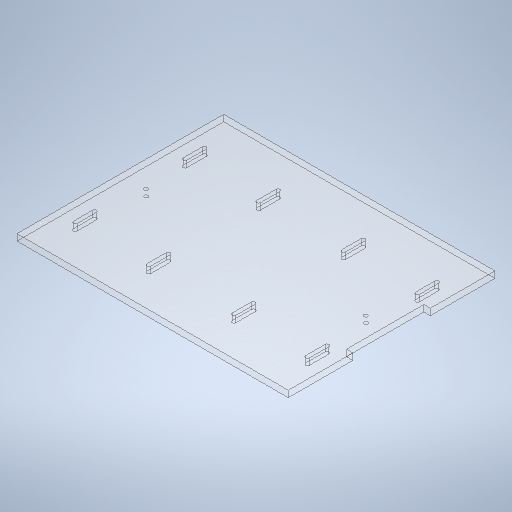
# Autodesk Inventor part: base_2
Saved by Autodesk Inventor 2025.3 (Build 293356030, 356C)
## iProperties
Created: 2026-06-26
Part Number: base_2
Material: Acrylic
Document SubType Name: Modeling
Designer: user
Density: 1.188 g/cm^3
Appearance: Transparent - Clear
Author: user
Autodesk Inventor part; units mm, degrees
ref_plane "YZ Plane" through (0, 0, 0) normal (1, 0, 0) x (0, 1, 0)
ref_plane "XZ Plane" through (0, 0, 0) normal (0, 1, 0) x (-1, 0, 0)
ref_plane "XY Plane" through (0, 0, 0) normal (0, 0, 1) x (1, 0, 0)
sketch "Sketch1" plane through (0, 0, 0) normal (0, 1, 0) x (-1, 0, 0)
  line L0 (0, 0) -> (-210, 0)
  line L1 (-210, 0) -> (-210, -160)
  line L2 (-210, -160) -> (0, -160)
  line L3 (75, -80) -> (-210, -80) construction
  line L4 (-105, 0) -> (-105, -160) construction
  line L5 (-43.5, 0) -> (-43.5, -160) construction
  line L6 (-133, 0) -> (-133, -160) construction
  line L7 (-15, -130) -> (-15, -115) construction
  line L8 (-15, -130) -> (-15, -115) construction
  line L9 (-13.5, -130) -> (-13.5, -115)
  line L10 (-16.5, -115) -> (-16.5, -130)
  arc A0 (-16.5, -130) -> (-13.5, -130) centre (-15, -130) ccw
  arc A1 (-13.5, -115) -> (-16.5, -115) centre (-15, -115) ccw
  line L11 (-72, -130) -> (-72, -115) construction
  line L12 (-72, -130) -> (-72, -115) construction
  line L13 (-73.5, -130) -> (-73.5, -115)
  line L14 (-70.5, -115) -> (-70.5, -130)
  arc A2 (-73.5, -130) -> (-70.5, -130) centre (-72, -130) ccw
  arc A3 (-70.5, -115) -> (-73.5, -115) centre (-72, -115) ccw
  line L15 (-125, -160) -> (-85, -160)
  line L16 (-85, -160) -> (-85, -155)
  line L17 (-85, -155) -> (-125, -155)
  line L18 (-125, -155) -> (-125, -160)
  line L19 (-195, -130) -> (-195, -115) construction
  line L20 (-195, -130) -> (-195, -115) construction
  line L21 (-196.5, -130) -> (-196.5, -115)
  line L22 (-193.5, -115) -> (-193.5, -130)
  arc A4 (-196.5, -130) -> (-193.5, -130) centre (-195, -130) ccw
  arc A5 (-193.5, -115) -> (-196.5, -115) centre (-195, -115) ccw
  line L23 (-139.5, -115) -> (-139.5, -130)
  line L24 (-138, -130) -> (-138, -115) construction
  line L25 (-136.5, -130) -> (-136.5, -115)
  arc A6 (-139.5, -130) -> (-136.5, -130) centre (-138, -130) ccw
  line L26 (-138, -130) -> (-138, -115) construction
  arc A7 (-136.5, -115) -> (-139.5, -115) centre (-138, -115) ccw
  line L27 (-105, -160) -> (-105, 0) construction
  line L28 (-15, -30) -> (-15, -45) construction
  line L29 (-15, -30) -> (-15, -45) construction
  line L30 (-13.5, -30) -> (-13.5, -45)
  line L31 (-16.5, -45) -> (-16.5, -30)
  arc A8 (-13.5, -30) -> (-16.5, -30) centre (-15, -30) ccw
  arc A9 (-16.5, -45) -> (-13.5, -45) centre (-15, -45) ccw
  line L32 (-70.5, -45) -> (-70.5, -30)
  line L33 (-72, -30) -> (-72, -45) construction
  line L34 (-73.5, -30) -> (-73.5, -45)
  arc A10 (-70.5, -30) -> (-73.5, -30) centre (-72, -30) ccw
  line L35 (-72, -30) -> (-72, -45) construction
  arc A11 (-73.5, -45) -> (-70.5, -45) centre (-72, -45) ccw
  line L36 (-125, 0) -> (-85, 0)
  line L37 (-85, 0) -> (-85, -5)
  line L38 (-85, -5) -> (-125, -5)
  line L39 (-125, -5) -> (-125, 0)
  arc A12 (-193.5, -30) -> (-196.5, -30) centre (-195, -30) ccw
  line L40 (-193.5, -45) -> (-193.5, -30)
  line L41 (-195, -30) -> (-195, -45) construction
  line L42 (-195, -30) -> (-195, -45) construction
  arc A13 (-196.5, -45) -> (-193.5, -45) centre (-195, -45) ccw
  line L43 (-196.5, -30) -> (-196.5, -45)
  line L44 (-139.5, -45) -> (-139.5, -30)
  line L45 (-138, -30) -> (-138, -45) construction
  line L46 (-138, -30) -> (-138, -45) construction
  arc A14 (-139.5, -45) -> (-136.5, -45) centre (-138, -45) ccw
  line L47 (-136.5, -30) -> (-136.5, -45)
  arc A15 (-136.5, -30) -> (-139.5, -30) centre (-138, -30) ccw
  line L48 (-210, -12.5) -> (-210, -62.5)
  line L49 (-210, -62.5) -> (-210, -110)
  line L50 (-210, -110) -> (-205, -110)
  line L51 (-205, -110) -> (-205, -50)
  line L52 (-205, -50) -> (-210, -50)
  line L53 (-210, -50) -> (-210, -12.5)
  line L54 (0, -160) -> (0, 0)
  point P0 (-15, -122.5)
  point P1 (-72, -122.5)
  point P2 (-195, -122.5)
  point P3 (-138, -122.5)
  point P4 (-15, -37.5)
  point P5 (-72, -37.5)
  point P6 (-195, -37.5)
  point P7 (-138, -37.5)
  point P8 (-72, -122.5)
  point P9 (-15, -122.5)
  point P10 (-125, -160)
  point P11 (-85, -160)
  point P12 (-85, 0)
  point P13 (-125, 0)
  point P14 (-195, -122.5)
  dimension "d2" = 15
  dimension "d4" = 30
  dimension "d6" = 1.5
  dimension "d9" = 40
  dimension "d13" = 0
  dimension "d14" = 5
  dimension "d16" = 20
  dimension "d22" = 5
  dimension "d26" = 30
  dimension "d27" = 30
  dimension "d28" = 0
  dimension "d30" = 160
  dimension "d32" = 57
  dimension "d56" = 15
  dimension "d57" = 210
  constraints: 126 end point, 55 symmetric about line, 32 point on circle, 16 centre point, 7 midpoint, 5 equal length, 5 perpendicular, 5 point on line, 4 tangent, 2 horizontal, 1 vertical, 14 other
  measures "d2" distance of L7.start L7.end
  measures "d4" distance from line of L2 L7.start
  measures "d6" radius of A0
  measures "d9" distance of L17.end L16.end
  measures "d13" distance between parallel lines of L2 L15
  measures "d14" distance between parallel lines of L17 L15
  measures "d16" distance between parallel lines of L4 L18
  measures "d22" distance between parallel lines of L49 L51
  measures "d26" distance between parallel lines of L3 L52
  measures "d27" distance between parallel lines of L3 L50
  measures "d28" distance between parallel lines of L1 L48
  measures "d30" distance between parallel lines of L0 L2
  measures "d32" distance of point (-72, -122.5) point (-15, -122.5)
  measures "d56" distance from line of L1 point (-195, -122.5)
  measures "d57" distance between parallel lines of L1 L54
extrude "Extrusion1" add sketch "Sketch1" along normal blind 5 contours L54 L2 L16 L17 L18 L1 L50 L51 L52 L0 L39 L38 L37 | L37 L38 L39 L0 | L2 L18 L17 L16
sketch "Sketch4" plane through (0, 5, 0) normal (0, 1, 0) x (1, 0, 0)
  line L0 (0, 0) -> (210, 0) projected
  line L1 (0, 160) -> (0, 0) projected
  point P0 (20, 80)
  dimension "d76" = 80
  dimension "d77" = 20
  measures "d76" distance from line of L0 point (20, 80)
  measures "d77" distance from line of L1 point (20, 80)
hole "Hole3" at (20, 5, -80) direction (0, -1, 0) diameter 3 end through all
sketch "Sketch5" plane through (0, 5, 0) normal (0, 1, 0) x (1, 0, 0)
  line L0 (205, 50) -> (205, 110) projected
  point P0 (0, 0)
  point P1 (190, 80)
  dimension "d85" = 15
  dimension "d86" = 30
  measures "d85" distance from line of L0 point (190, 80)
  measures "d86" vertical distance of point (190, 80) L0.end
hole "Hole4" at (190, 5, -80) direction (0, -1, 0) diameter 3 end through all
body "Solid1"
